Autodesk Inventor part; units mm, degrees
(part 2 of 2)
sketch "Sketch39" plane through (0, 15, 0) normal (0, 1, 0) x (1, 0, 0)
  circle A0 centre (1.2218, -51.2393) radius 1.65 projected
  circle A1 centre (75, -20) radius 1.65 projected
  circle A2 centre (75, 20) radius 1.65 projected
  circle A3 centre (1.2218, 51.2393) radius 1.65 projected
  circle A4 centre (50, -41.2393) radius 1.65 projected
  circle A5 centre (50, 41.4252) radius 1.65 projected
  arc A6 (-52, -67.2384) -> (-18.7782, -82.8998) centre (0, 0) ccw projected
  line L0 (-52, -67.2384) -> (-52, 67.2384) projected
  arc A7 (-18.7782, 82.8998) -> (-52, 67.2384) centre (0, 0) ccw projected
  line L1 (-18.7782, 82.8998) -> (-18.7782, -82.8998) projected
  circle A8 centre (-8.7782, 43.7683) radius 1.6079 projected
  circle A9 centre (-8.778, -38.7103) radius 1.6079 projected
  circle A10 centre (1.2218, -41.2393) radius 1.65 projected
  circle A11 centre (1.2218, 41.2393) radius 1.65 projected
  line L2 (-28.2493, 88.8562) -> (-25.8738, 89.6874) projected
  line L3 (-25.8738, 89.6874) -> (-24.5197, 85.8175) projected
  line L4 (-24.5197, 85.8175) -> (-34.3361, 82.3826) projected
  line L5 (-34.3361, 82.3826) -> (-35.6902, 86.2525) projected
  line L6 (-35.6902, 86.2525) -> (-33.3147, 87.0837) projected
  arc A12 (-28.2493, 88.8562) -> (-33.3147, 87.0837) centre (-30.4187, 86.9317) ccw projected
  line L7 (30.0353, 88.2685) -> (32.4402, 87.5267) projected
  line L8 (32.4402, 87.5267) -> (31.2317, 83.6088) projected
  line L9 (31.2317, 83.6088) -> (21.2937, 86.6743) projected
  line L10 (21.2937, 86.6743) -> (22.5022, 90.5921) projected
  line L11 (22.5022, 90.5921) -> (24.9071, 89.8503) projected
  arc A13 (30.0353, 88.2685) -> (24.9071, 89.8503) centre (27.147, 88.0083) ccw projected
  line L12 (79.29, 49.114) -> (80.6765, 47.0136) projected
  line L13 (80.6765, 47.0136) -> (77.2547, 44.7549) projected
  line L14 (77.2547, 44.7549) -> (71.5254, 53.4345) projected
  line L15 (71.5254, 53.4345) -> (74.9472, 55.6931) projected
  line L16 (74.9472, 55.6931) -> (76.3336, 53.5927) projected
  arc A14 (79.29, 49.114) -> (76.3336, 53.5927) centre (76.8938, 50.7474) ccw projected
  line L17 (93.2, -2.6833) -> (93.2, -5.2) projected
  line L18 (93.2, -5.2) -> (89.1, -5.2) projected
  line L19 (89.1, -5.2) -> (89.1, 5.2) projected
  line L20 (89.1, 5.2) -> (93.2, 5.2) projected
  line L21 (93.2, 5.2) -> (93.2, 2.6833) projected
  arc A15 (93.2, -2.6833) -> (93.2, 2.6833) centre (92.1, 0) ccw projected
  line L22 (76.6444, -54.0482) -> (75.2579, -56.1486) projected
  line L23 (75.2579, -56.1486) -> (71.8362, -53.8899) projected
  line L24 (71.8362, -53.8899) -> (77.5655, -45.2103) projected
  line L25 (77.5655, -45.2103) -> (80.9873, -47.469) projected
  line L26 (80.9873, -47.469) -> (79.6008, -49.5694) projected
  arc A16 (76.6444, -54.0482) -> (79.6008, -49.5694) centre (77.2046, -51.2028) ccw projected
  line L27 (24.9071, -89.8503) -> (22.5022, -90.5921) projected
  line L28 (22.5022, -90.5921) -> (21.2937, -86.6743) projected
  line L29 (21.2937, -86.6743) -> (31.2317, -83.6088) projected
  line L30 (31.2317, -83.6088) -> (32.4402, -87.5267) projected
  line L31 (32.4402, -87.5267) -> (30.0353, -88.2685) projected
  arc A17 (24.9071, -89.8503) -> (30.0353, -88.2685) centre (27.147, -88.0083) ccw projected
  line L32 (-33.3147, -87.0837) -> (-35.6902, -86.2525) projected
  line L33 (-35.6902, -86.2525) -> (-34.3361, -82.3826) projected
  line L34 (-34.3361, -82.3826) -> (-24.5197, -85.8175) projected
  line L35 (-24.5197, -85.8175) -> (-25.8738, -89.6874) projected
  line L36 (-25.8738, -89.6874) -> (-28.2493, -88.8562) projected
  arc A18 (-33.3147, -87.0837) -> (-28.2493, -88.8562) centre (-30.4187, -86.9317) ccw projected
  line L37 (-68.5526, -41.4252) -> (-65.0019, -39.3752) projected
  line L38 (-65.0019, -39.3752) -> (-59.8019, -48.3819) projected
  line L39 (-59.8019, -48.3819) -> (-63.3526, -50.4319) projected
  line L40 (-63.3526, -50.4319) -> (-64.611, -48.2524) projected
  arc A19 (-67.2943, -43.6048) -> (-64.611, -48.2524) centre (-65, -45.3786) ccw projected
  line L41 (-67.2943, -43.6048) -> (-68.5526, -41.4252) projected
  line L42 (-64.7167, 27.997) -> (-60.7564, 26.9359) projected
  line L43 (-60.7564, 26.9359) -> (-63.4481, 16.8902) projected
  line L44 (-63.4481, 16.8902) -> (-67.4084, 17.9514) projected
  line L45 (-67.4084, 17.9514) -> (-66.757, 20.3823) projected
  arc A20 (-65.368, 25.5661) -> (-66.757, 20.3823) centre (-65, 22.6895) ccw projected
  line L46 (-65.368, 25.5661) -> (-64.7167, 27.997) projected
  line L47 (-66.1, 5.2) -> (-62, 5.2) projected
  line L48 (-62, 5.2) -> (-62, -5.2) projected
  line L49 (-62, -5.2) -> (-66.1, -5.2) projected
  line L50 (-66.1, -5.2) -> (-66.1, -2.6833) projected
  arc A21 (-66.1, 2.6833) -> (-66.1, -2.6833) centre (-65, 0) ccw projected
  line L51 (-66.1, 2.6833) -> (-66.1, 5.2) projected
  line L52 (-67.4084, -17.9514) -> (-63.4481, -16.8902) projected
  line L53 (-63.4481, -16.8902) -> (-60.7564, -26.9359) projected
  line L54 (-60.7564, -26.9359) -> (-64.7167, -27.997) projected
  line L55 (-64.7167, -27.997) -> (-65.368, -25.5661) projected
  arc A22 (-66.757, -20.3823) -> (-65.368, -25.5661) centre (-65, -22.6895) ccw projected
  line L56 (-66.757, -20.3823) -> (-67.4084, -17.9514) projected
  line L57 (-63.3526, 50.4319) -> (-59.8019, 48.3819) projected
  line L58 (-59.8019, 48.3819) -> (-65.0019, 39.3752) projected
  line L59 (-65.0019, 39.3752) -> (-68.5526, 41.4252) projected
  line L60 (-68.5526, 41.4252) -> (-67.2943, 43.6048) projected
  arc A23 (-64.611, 48.2524) -> (-67.2943, 43.6048) centre (-65, 45.3786) ccw projected
  line L61 (-64.611, 48.2524) -> (-63.3526, 50.4319) projected
  line L62 (-60.862, -70.775) -> (-58.3661, -67.5222) projected
  line L63 (-58.3661, -67.5222) -> (-50.1152, -73.8533) projected
  line L64 (-50.1152, -73.8533) -> (-52.6111, -77.1061) projected
  line L65 (-52.6111, -77.1061) -> (-54.6078, -75.574) projected
  arc A24 (-58.8654, -72.3071) -> (-54.6078, -75.574) centre (-56.0669, -73.0678) ccw projected
  line L66 (-58.8654, -72.3071) -> (-60.862, -70.775) projected
  line L67 (-4.4255, -93.1335) -> (-6.9418, -93.0865) projected
  line L68 (-6.9418, -93.0865) -> (-6.8652, -88.9872) projected
  line L69 (-6.8652, -88.9872) -> (3.533, -89.1817) projected
  line L70 (3.533, -89.1817) -> (3.4564, -93.2809) projected
  line L71 (3.4564, -93.2809) -> (0.9401, -93.2339) projected
  arc A25 (-4.4255, -93.1335) -> (0.9401, -93.2339) centre (-1.7222, -92.0839) ccw projected
  line L72 (51.7438, -77.563) -> (49.6912, -79.0194) projected
  line L73 (49.6912, -79.0194) -> (47.3187, -75.6756) projected
  line L74 (47.3187, -75.6756) -> (55.8005, -69.6574) projected
  line L75 (55.8005, -69.6574) -> (58.1731, -73.0012) projected
  line L76 (58.1731, -73.0012) -> (56.1205, -74.4575) projected
  arc A26 (51.7438, -77.563) -> (56.1205, -74.4575) centre (53.2956, -75.1132) ccw projected
  line L77 (87.6914, -31.6805) -> (86.9048, -34.0711) projected
  line L78 (86.9048, -34.0711) -> (83.0102, -32.7896) projected
  line L79 (83.0102, -32.7896) -> (86.2609, -22.9107) projected
  line L80 (86.2609, -22.9107) -> (90.1555, -24.1922) projected
  line L81 (90.1555, -24.1922) -> (89.3689, -26.5829) projected
  arc A27 (87.6914, -31.6805) -> (89.3689, -26.5829) centre (87.4853, -28.7879) ccw projected
  line L82 (89.3689, 26.5829) -> (90.1555, 24.1922) projected
  line L83 (90.1555, 24.1922) -> (86.2609, 22.9107) projected
  line L84 (86.2609, 22.9107) -> (83.0102, 32.7896) projected
  line L85 (83.0102, 32.7896) -> (86.9048, 34.0711) projected
  line L86 (86.9048, 34.0711) -> (87.6914, 31.6805) projected
  arc A28 (89.3689, 26.5829) -> (87.6914, 31.6805) centre (87.4853, 28.7879) ccw projected
  line L87 (56.1205, 74.4575) -> (58.1731, 73.0012) projected
  line L88 (58.1731, 73.0012) -> (55.8005, 69.6574) projected
  line L89 (55.8005, 69.6574) -> (47.3187, 75.6756) projected
  line L90 (47.3187, 75.6756) -> (49.6912, 79.0194) projected
  line L91 (49.6912, 79.0194) -> (51.7438, 77.563) projected
  arc A29 (56.1205, 74.4575) -> (51.7438, 77.563) centre (53.2956, 75.1132) ccw projected
  line L92 (0.9401, 93.2339) -> (3.4564, 93.2809) projected
  line L93 (3.4564, 93.2809) -> (3.533, 89.1817) projected
  line L94 (3.533, 89.1817) -> (-6.8652, 88.9872) projected
  line L95 (-6.8652, 88.9872) -> (-6.9418, 93.0865) projected
  line L96 (-6.9418, 93.0865) -> (-4.4255, 93.1335) projected
  arc A30 (0.9401, 93.2339) -> (-4.4255, 93.1335) centre (-1.7222, 92.0839) ccw projected
  line L97 (-54.6078, 75.574) -> (-52.6111, 77.1061) projected
  line L98 (-52.6111, 77.1061) -> (-50.1152, 73.8533) projected
  line L99 (-50.1152, 73.8533) -> (-58.3661, 67.5222) projected
  line L100 (-58.3661, 67.5222) -> (-60.862, 70.775) projected
  line L101 (-60.862, 70.775) -> (-58.8654, 72.3071) projected
  arc A31 (-54.6078, 75.574) -> (-58.8654, 72.3071) centre (-56.0669, 73.0678) ccw projected
  circle A32 centre (-57, -37.4412) radius 1.25 projected
  circle A33 centre (-57, 37.4412) radius 1.25 projected
  circle A34 centre (-69.5802, -56.8899) radius 3 projected
  circle A35 centre (-69.5802, 56.8899) radius 3 projected
  circle A36 centre (71.6532, 61.1111) radius 3 projected
  circle A37 centre (71.6532, -61.1111) radius 3 projected
  line L102 (6.2218, -84.772) -> (6.2218, 84.772) projected
  arc A38 (45, 72.111) -> (6.2218, 84.772) centre (0, 0) ccw projected
  line L103 (45, 72.111) -> (45, -72.111) projected
  arc A39 (6.2218, -84.772) -> (45, -72.111) centre (0, 0) ccw projected
  arc A40 (-85, -52.6783) -> (-85, 52.6783) centre (0, 0) ccw projected
  line L104 (-18.7782, 82.8998) -> (6.2218, 82.8998)
  line L105 (6.2218, -84.772) -> (6.2218, 84.772) projected
  line L106 (-18.7782, 83.6088) -> (-18.7782, 63.6088)
  line L107 (-18.7782, 82.8998) -> (-18.7782, -82.8998) projected
  line L108 (-18.7782, 63.6088) -> (6.2218, 63.6088)
  line L109 (6.2218, 63.6088) -> (6.2218, 82.8998)
  line L110 (-85, 52.6783) -> (-85, 47.6783) projected
  line L111 (-85, -47.6783) -> (-85, -52.6783) projected
  line L112 (-70, 0) -> (-85, -47.6783) projected
  line L113 (-85, 47.6783) -> (-70, 0) projected
  dimension "d78" = 10.4
  dimension "d79" = 4.1
  dimension "d243" = 20
  constraints: 8 end point, 3 point on line, 1 collinear, 1 horizontal, 1 perpendicular
  measures "d243" distance of L106.start L106.end
extrude "Extrusion37" add sketch "Sketch39" along normal blind 25 contours L1 L104 L102 L108
sketch "Sketch40" plane through (-18.7782, 15, -63.6088) normal (0, 0, 1) x (1, 0, 0)
  line L0 (0, -5) -> (0, 0) projected
  line L1 (2.25, 1) -> (22.75, 1)
  line L2 (22.75, 1) -> (22.75, 24)
  line L3 (22.75, 24) -> (2.25, 24)
  line L4 (2.25, 24) -> (2.25, 1)
  line L5 (2.25, 1) -> (22.75, 24) construction
  line L6 (22.75, 1) -> (2.25, 24) construction
  line L7 (25, 0) -> (25, 25) projected
  point P0 (18.7782, -15)
  point P1 (0, 25)
  point P2 (12.5, 12.5)
  dimension "d246" = 20.5
  dimension "d247" = 23
  constraints: 12 end point, 2 midpoint, 2 parallel, 2 perpendicular
  measures "d246" distance of L1.start L1.end
  measures "d247" distance of L2.end L1.end
extrude "Extrusion38" cut sketch "Sketch40" against normal blind 5
sketch "Sketch41" plane through (-18.7782, 15, -68.6088) normal (0, 0, 1) x (1, 0, 0)
  line L0 (22.75, 1) -> (2.25, 1) projected
  line L1 (22.75, 24) -> (22.75, 1) projected
  line L2 (2.25, 24) -> (22.75, 24) projected
  line L3 (2.25, 1) -> (2.25, 24) projected
  line L4 (22.75, 1) -> (2.25, 1)
  circle A0 centre (13.7, 12.5) radius 8.5
  line L5 (22.75, 1) -> (22.45, 1)
  line L6 (22.75, 1) -> (2.25, 1) projected
  line L7 (22.45, 1) -> (22.45, 1.45)
  line L8 (22.45, 1.45) -> (20, 1.45)
  line L9 (20, 1.45) -> (20, 3.9)
  line L10 (20, 3.9) -> (7.4, 3.9)
  line L11 (13.7, 3.9) -> (13.7, 12.5)
  line L12 (13.7, 3.9) -> (22.3, 3.9) construction
  point P0 (18.7782, -15)
  dimension "d250" = 17
  dimension "d272" = 0.3
  dimension "d273" = 0.45
  dimension "d274" = 2.45
  dimension "d275" = 2.45
  dimension "d276" = 12.6
  dimension "d277" = 90
  constraints: 16 end point, 5 perpendicular, 1 centre point, 1 collinear, 1 horizontal, 1 midpoint, 1 point on line
  measures "d250" diameter of A0
  measures "d272" distance of L0.start L5.end
  measures "d273" distance of L5.end L7.end
  measures "d274" distance of L7.end L8.end
  measures "d275" distance of L8.end L9.end
  measures "d276" distance of L9.end L10.end
  measures "d277" angle of L12 L11
extrude "Extrusion39" cut sketch "Sketch41" against normal blind 48.5 contours A0
sketch "Sketch42" plane through (-18.7782, 15, -68.6088) normal (0, 0, 1) x (1, 0, 0)
  circle A0 centre (13.7, 12.5) radius 8.5 projected
  line L0 (22.75, 1) -> (2.25, 1) projected
  line L1 (22.75, 24) -> (22.75, 1) projected
  line L2 (2.25, 24) -> (22.75, 24) projected
  line L3 (2.25, 1) -> (2.25, 24) projected
  line L4 (22.75, 1) -> (22.75, 1.45)
  line L5 (22.75, 24) -> (22.75, 1) projected
  line L6 (22.75, 1.45) -> (22.75, 3.99)
  line L7 (2.25, 1) -> (2.25, 24) projected
  line L8 (2.25, 4) -> (2.55, 4)
  line L9 (22.75, 24) -> (22.75, 23.55)
  line L10 (22.45, 1.45) -> (2.55, 1.45)
  line L11 (2.55, 1.45) -> (2.55, 23.55)
  line L12 (2.55, 23.55) -> (22.45, 23.55)
  line L13 (22.45, 23.55) -> (22.45, 1.45)
  line L14 (22.45, 1.45) -> (22.45, 3.99)
  line L15 (22.45, 3.99) -> (19.91, 3.99)
  line L16 (19.91, 3.99) -> (7.31, 3.99)
  line L17 (7.31, 3.99) -> (7.31, 20.99)
  line L18 (7.31, 20.99) -> (19.91, 20.99)
  circle A1 centre (7.31, 20.99) radius 1.25
  circle A2 centre (19.91, 3.99) radius 1.25
  point P0 (18.7782, -15)
  dimension "d253" = 0.45
  dimension "d254" = 2.54
  dimension "d261" = 0.3
  dimension "d262" = 0.45
  dimension "d263" = 0.3
  dimension "d264" = 2.54
  dimension "d265" = 2.54
  dimension "d266" = 12.6
  dimension "d267" = 17
  dimension "d268" = 2.5
  dimension "d269" = 2.5
  constraints: 26 end point, 6 perpendicular, 6 point on line, 2 centre point, 2 coincident, 1 parallel
  measures "d253" distance of L0.start L4.end
  measures "d254" distance of L4.end L6.end
  measures "d261" distance of L8.start L8.end
  measures "d262" distance of L1.start L9.end
  measures "d263" distance of L4.end L10.start
  measures "d264" distance of L10.start L14.end
  measures "d265" distance of L14.end L15.end
  measures "d266" distance of L15.end L16.end
  measures "d267" distance of L16.end L17.end
  measures "d268" diameter of A1
  measures "d269" diameter of A2
extrude "Extrusion40" cut sketch "Sketch42" against normal blind 10 contours A1 L17 L18 | L18 L17 A1 | A2 L16 L15 | L15 L16 A2
sketch "Sketch43" plane through (0, 15, 0) normal (0, 1, 0) x (1, 0, 0)
  line L0 (-18.7782, -82.8998) -> (6.2218, -82.8998)
  line L1 (6.2218, -84.772) -> (6.2218, 63.6088) projected
  line L2 (-18.7782, -82.8998) -> (-18.7782, -62.8998)
  line L3 (-18.7782, -82.8998) -> (-18.7782, 82.8998) projected
  line L4 (6.2218, -82.8998) -> (6.2218, -62.8998)
  line L5 (6.2218, -62.8998) -> (-18.7782, -62.8998)
  line L6 (-18.7782, 63.6088) -> (-18.7782, -82.8998) projected
  point P0 (0, 0)
  dimension "d278" = 20
  constraints: 8 end point, 3 point on line, 1 horizontal, 1 perpendicular
  measures "d278" distance of L0.start L2.end
extrude "Extrusion41" add sketch "Sketch43" along normal blind 25
sketch "Sketch44" plane through (6.2218, 15, 62.8998) normal (0, 0, -1) x (-1, 0, 0)
  line L0 (2.25, 1) -> (22.75, 1) projected
  line L1 (2.25, 24) -> (2.25, 1) projected
  line L2 (22.75, 24) -> (2.25, 24) projected
  line L3 (22.75, 1) -> (22.75, 24) projected
  point P0 (6.2218, -15)
extrude "Extrusion42" cut sketch "Sketch44" against normal blind 5
sketch "Sketch45" plane through (6.2218, 15, 67.8998) normal (0, 0, -1) x (-1, 0, 0)
  line L0 (22.75, 1) -> (2.25, 1) projected
  line L1 (22.75, 24) -> (22.75, 1) projected
  line L2 (2.25, 24) -> (22.75, 24) projected
  line L3 (2.25, 1) -> (2.25, 24) projected
  line L4 (22.75, 1) -> (22.75, 1.45)
  line L5 (22.75, 24) -> (22.75, 1) projected
  line L6 (22.45, 1.45) -> (24.9, 1.45) construction
  circle A0 centre (13.7, 12.5) radius 8.5
  circle A1 centre (20, 3.9) radius 1.25
  circle A2 centre (7.4, 20.9) radius 1.25
  point P0 (6.2218, -15)
  dimension "d283" = 0.45
  dimension "d284" = 0.3
  dimension "d292" = 2.5
  dimension "d295" = 2.5
  constraints: 4 end point, 3 centre point, 1 horizontal, 1 point on line
  measures "d283" distance of L0.start L4.end
  measures "d284" distance of L4.end L6.start
  measures "d292" diameter of A1
  measures "d295" diameter of A2
extrude "Extrusion43" cut sketch "Sketch45" against normal through all contours A0
sketch "Sketch46" plane through (6.2218, 15, 67.8998) normal (0, 0, -1) x (-1, 0, 0)
  line L0 (22.75, 1) -> (2.25, 1)
  line L1 (22.75, 24) -> (22.75, 1)
  line L2 (2.25, 24) -> (22.75, 24)
  line L3 (2.25, 1) -> (2.25, 24)
  line L4 (22.75, 1) -> (22.75, 1.45)
  line L5 (22.75, 24) -> (22.75, 1)
  line L6 (22.45, 1.45) -> (24.9, 1.45) construction
  circle A0 centre (13.7, 12.5) radius 8.5
  circle A1 centre (20, 3.9) radius 1.25
  circle A2 centre (7.4, 20.9) radius 1.25
  point P0 (6.2218, -15)
  dimension "d298" = 0.45
  dimension "d299" = 0.3
  dimension "d300" = 2.5
  dimension "d301" = 2.5
  constraints: 14 end point, 3 centre point, 1 horizontal, 1 point on line
  measures "d298" distance of L0.start L4.end
  measures "d299" distance of L4.end L6.start
  measures "d300" diameter of A1
  measures "d301" diameter of A2
extrude "Extrusion44" cut sketch "Sketch46" against normal blind 10 contours A1 | A2
sketch "Sketch47" plane through (0, 15, 0) normal (0, 1, 0) x (1, 0, 0)
  circle A0 centre (75, -20) radius 1.65 projected
  circle A1 centre (75, 20) radius 1.65 projected
  circle A2 centre (50, -41.2393) radius 1.65 projected
  circle A3 centre (50, 41.4252) radius 1.65 projected
  line L0 (-28.2493, 88.8562) -> (-25.8738, 89.6874) projected
  line L1 (-25.8738, 89.6874) -> (-24.5197, 85.8175) projected
  line L2 (-24.5197, 85.8175) -> (-34.3361, 82.3826) projected
  line L3 (-34.3361, 82.3826) -> (-35.6902, 86.2525) projected
  line L4 (-35.6902, 86.2525) -> (-33.3147, 87.0837) projected
  arc A4 (-28.2493, 88.8562) -> (-33.3147, 87.0837) centre (-30.4187, 86.9317) ccw projected
  line L5 (30.0353, 88.2685) -> (32.4402, 87.5267) projected
  line L6 (32.4402, 87.5267) -> (31.2317, 83.6088) projected
  line L7 (31.2317, 83.6088) -> (21.2937, 86.6743) projected
  line L8 (21.2937, 86.6743) -> (22.5022, 90.5921) projected
  line L9 (22.5022, 90.5921) -> (24.9071, 89.8503) projected
  arc A5 (30.0353, 88.2685) -> (24.9071, 89.8503) centre (27.147, 88.0083) ccw projected
  line L10 (79.29, 49.114) -> (80.6765, 47.0136) projected
  line L11 (80.6765, 47.0136) -> (77.2547, 44.7549) projected
  line L12 (77.2547, 44.7549) -> (71.5254, 53.4345) projected
  line L13 (71.5254, 53.4345) -> (74.9472, 55.6931) projected
  line L14 (74.9472, 55.6931) -> (76.3336, 53.5927) projected
  arc A6 (79.29, 49.114) -> (76.3336, 53.5927) centre (76.8938, 50.7474) ccw projected
  line L15 (93.2, -2.6833) -> (93.2, -5.2) projected
  line L16 (93.2, -5.2) -> (89.1, -5.2) projected
  line L17 (89.1, -5.2) -> (89.1, 5.2) projected
  line L18 (89.1, 5.2) -> (93.2, 5.2) projected
  line L19 (93.2, 5.2) -> (93.2, 2.6833) projected
  arc A7 (93.2, -2.6833) -> (93.2, 2.6833) centre (92.1, 0) ccw projected
  line L20 (76.6444, -54.0482) -> (75.2579, -56.1486) projected
  line L21 (75.2579, -56.1486) -> (71.8362, -53.8899) projected
  line L22 (71.8362, -53.8899) -> (77.5655, -45.2103) projected
  line L23 (77.5655, -45.2103) -> (80.9873, -47.469) projected
  line L24 (80.9873, -47.469) -> (79.6008, -49.5694) projected
  arc A8 (76.6444, -54.0482) -> (79.6008, -49.5694) centre (77.2046, -51.2028) ccw projected
  line L25 (24.9071, -89.8503) -> (22.5022, -90.5921) projected
  line L26 (22.5022, -90.5921) -> (21.2937, -86.6743) projected
  line L27 (21.2937, -86.6743) -> (31.2317, -83.6088) projected
  line L28 (31.2317, -83.6088) -> (32.4402, -87.5267) projected
  line L29 (32.4402, -87.5267) -> (30.0353, -88.2685) projected
  arc A9 (24.9071, -89.8503) -> (30.0353, -88.2685) centre (27.147, -88.0083) ccw projected
  line L30 (-33.3147, -87.0837) -> (-35.6902, -86.2525) projected
  line L31 (-35.6902, -86.2525) -> (-34.3361, -82.3826) projected
  line L32 (-34.3361, -82.3826) -> (-24.5197, -85.8175) projected
  line L33 (-24.5197, -85.8175) -> (-25.8738, -89.6874) projected
  line L34 (-25.8738, -89.6874) -> (-28.2493, -88.8562) projected
  arc A10 (-33.3147, -87.0837) -> (-28.2493, -88.8562) centre (-30.4187, -86.9317) ccw projected
  line L35 (-68.5526, -41.4252) -> (-65.0019, -39.3752) projected
  line L36 (-65.0019, -39.3752) -> (-59.8019, -48.3819) projected
  line L37 (-59.8019, -48.3819) -> (-63.3526, -50.4319) projected
  line L38 (-63.3526, -50.4319) -> (-64.611, -48.2524) projected
  arc A11 (-67.2943, -43.6048) -> (-64.611, -48.2524) centre (-65, -45.3786) ccw projected
  line L39 (-67.2943, -43.6048) -> (-68.5526, -41.4252) projected
  line L40 (-64.7167, 27.997) -> (-60.7564, 26.9359) projected
  line L41 (-60.7564, 26.9359) -> (-63.4481, 16.8902) projected
  line L42 (-63.4481, 16.8902) -> (-67.4084, 17.9514) projected
  line L43 (-67.4084, 17.9514) -> (-66.757, 20.3823) projected
  arc A12 (-65.368, 25.5661) -> (-66.757, 20.3823) centre (-65, 22.6895) ccw projected
  line L44 (-65.368, 25.5661) -> (-64.7167, 27.997) projected
  line L45 (-66.1, 5.2) -> (-62, 5.2) projected
  line L46 (-62, 5.2) -> (-62, -5.2) projected
  line L47 (-62, -5.2) -> (-66.1, -5.2) projected
  line L48 (-66.1, -5.2) -> (-66.1, -2.6833) projected
  arc A13 (-66.1, 2.6833) -> (-66.1, -2.6833) centre (-65, 0) ccw projected
  line L49 (-66.1, 2.6833) -> (-66.1, 5.2) projected
  line L50 (-67.4084, -17.9514) -> (-63.4481, -16.8902) projected
  line L51 (-63.4481, -16.8902) -> (-60.7564, -26.9359) projected
  line L52 (-60.7564, -26.9359) -> (-64.7167, -27.997) projected
  line L53 (-64.7167, -27.997) -> (-65.368, -25.5661) projected
  arc A14 (-66.757, -20.3823) -> (-65.368, -25.5661) centre (-65, -22.6895) ccw projected
  line L54 (-66.757, -20.3823) -> (-67.4084, -17.9514) projected
  line L55 (-63.3526, 50.4319) -> (-59.8019, 48.3819) projected
  line L56 (-59.8019, 48.3819) -> (-65.0019, 39.3752) projected
  line L57 (-65.0019, 39.3752) -> (-68.5526, 41.4252) projected
  line L58 (-68.5526, 41.4252) -> (-67.2943, 43.6048) projected
  arc A15 (-64.611, 48.2524) -> (-67.2943, 43.6048) centre (-65, 45.3786) ccw projected
  line L59 (-64.611, 48.2524) -> (-63.3526, 50.4319) projected
  line L60 (-60.862, -70.775) -> (-58.3661, -67.5222) projected
  line L61 (-58.3661, -67.5222) -> (-50.1152, -73.8533) projected
  line L62 (-50.1152, -73.8533) -> (-52.6111, -77.1061) projected
  line L63 (-52.6111, -77.1061) -> (-54.6078, -75.574) projected
  arc A16 (-58.8654, -72.3071) -> (-54.6078, -75.574) centre (-56.0669, -73.0678) ccw projected
  line L64 (-58.8654, -72.3071) -> (-60.862, -70.775) projected
  line L65 (-4.4255, -93.1335) -> (-6.9418, -93.0865) projected
  line L66 (-6.9418, -93.0865) -> (-6.8652, -88.9872) projected
  line L67 (-6.8652, -88.9872) -> (3.533, -89.1817) projected
  line L68 (3.533, -89.1817) -> (3.4564, -93.2809) projected
  line L69 (3.4564, -93.2809) -> (0.9401, -93.2339) projected
  arc A17 (-4.4255, -93.1335) -> (0.9401, -93.2339) centre (-1.7222, -92.0839) ccw projected
  line L70 (51.7438, -77.563) -> (49.6912, -79.0194) projected
  line L71 (49.6912, -79.0194) -> (47.3187, -75.6756) projected
  line L72 (47.3187, -75.6756) -> (55.8005, -69.6574) projected
  line L73 (55.8005, -69.6574) -> (58.1731, -73.0012) projected
  line L74 (58.1731, -73.0012) -> (56.1205, -74.4575) projected
  arc A18 (51.7438, -77.563) -> (56.1205, -74.4575) centre (53.2956, -75.1132) ccw projected
  line L75 (87.6914, -31.6805) -> (86.9048, -34.0711) projected
  line L76 (86.9048, -34.0711) -> (83.0102, -32.7896) projected
  line L77 (83.0102, -32.7896) -> (86.2609, -22.9107) projected
  line L78 (86.2609, -22.9107) -> (90.1555, -24.1922) projected
  line L79 (90.1555, -24.1922) -> (89.3689, -26.5829) projected
  arc A19 (87.6914, -31.6805) -> (89.3689, -26.5829) centre (87.4853, -28.7879) ccw projected
  line L80 (89.3689, 26.5829) -> (90.1555, 24.1922) projected
  line L81 (90.1555, 24.1922) -> (86.2609, 22.9107) projected
  line L82 (86.2609, 22.9107) -> (83.0102, 32.7896) projected
  line L83 (83.0102, 32.7896) -> (86.9048, 34.0711) projected
  line L84 (86.9048, 34.0711) -> (87.6914, 31.6805) projected
  arc A20 (89.3689, 26.5829) -> (87.6914, 31.6805) centre (87.4853, 28.7879) ccw projected
  line L85 (56.1205, 74.4575) -> (58.1731, 73.0012) projected
  line L86 (58.1731, 73.0012) -> (55.8005, 69.6574) projected
  line L87 (55.8005, 69.6574) -> (47.3187, 75.6756) projected
  line L88 (47.3187, 75.6756) -> (49.6912, 79.0194) projected
  line L89 (49.6912, 79.0194) -> (51.7438, 77.563) projected
  arc A21 (56.1205, 74.4575) -> (51.7438, 77.563) centre (53.2956, 75.1132) ccw projected
  line L90 (0.9401, 93.2339) -> (3.4564, 93.2809) projected
  line L91 (3.4564, 93.2809) -> (3.533, 89.1817) projected
  line L92 (3.533, 89.1817) -> (-6.8652, 88.9872) projected
  line L93 (-6.8652, 88.9872) -> (-6.9418, 93.0865) projected
  line L94 (-6.9418, 93.0865) -> (-4.4255, 93.1335) projected
  arc A22 (0.9401, 93.2339) -> (-4.4255, 93.1335) centre (-1.7222, 92.0839) ccw projected
  line L95 (-54.6078, 75.574) -> (-52.6111, 77.1061) projected
  line L96 (-52.6111, 77.1061) -> (-50.1152, 73.8533) projected
  line L97 (-50.1152, 73.8533) -> (-58.3661, 67.5222) projected
  line L98 (-58.3661, 67.5222) -> (-60.862, 70.775) projected
  line L99 (-60.862, 70.775) -> (-58.8654, 72.3071) projected
  arc A23 (-54.6078, 75.574) -> (-58.8654, 72.3071) centre (-56.0669, 73.0678) ccw projected
  circle A24 centre (-57, -37.4412) radius 1.25 projected
  circle A25 centre (-57, 37.4412) radius 1.25 projected
  circle A26 centre (-69.5802, -56.8899) radius 3 projected
  circle A27 centre (-69.5802, 56.8899) radius 3 projected
  circle A28 centre (71.6532, 61.1111) radius 3 projected
  circle A29 centre (71.6532, -61.1111) radius 3 projected
  arc A30 (-85, -52.6783) -> (-85, 52.6783) centre (0, 0) ccw projected
  line L100 (6.2218, -82.8998) -> (-18.7782, -82.8998) projected
  arc A31 (-52, -67.2384) -> (-18.7782, -82.8998) centre (0, 0) ccw projected
  line L101 (-52, -67.2384) -> (-52, 67.2384) projected
  arc A32 (-18.7782, 82.8998) -> (-52, 67.2384) centre (0, 0) ccw projected
  line L102 (-18.7782, 82.8998) -> (6.2218, 82.8998) projected
  line L103 (6.2218, 82.8998) -> (6.2218, 84.772) projected
  arc A33 (45, 72.111) -> (6.2218, 84.772) centre (0, 0) ccw projected
  line L104 (45, 72.111) -> (45, -72.111) projected
  arc A34 (6.2218, -84.772) -> (45, -72.111) centre (0, 0) ccw projected
  line L105 (6.2218, -84.772) -> (6.2218, -82.8998) projected
  line L106 (82, 0) -> (82, -12.5)
  line L107 (82, -12.5) -> (62, -12.5)
  line L108 (62, -12.5) -> (62, 12.5)
  line L109 (62, 12.5) -> (82, 12.5)
  line L110 (82, 12.5) -> (82, 0)
  line L111 (-85, 52.6783) -> (-85, 47.6783) projected
  line L112 (-85, -47.6783) -> (-85, -52.6783) projected
  line L113 (-70, 0) -> (-85, -47.6783) projected
  line L114 (-85, 47.6783) -> (-70, 0) projected
  dimension "d306" = 20
  dimension "d307" = 25
  constraints: 10 end point, 4 perpendicular, 1 point on line, 1 vertical
  measures "d306" distance of L106.end L107.end
  measures "d307" distance of L107.end L108.end
extrude "Extrusion45" add sketch "Sketch47" along normal blind 25 contours L106 L107 L108 L109 L110
sketch "Sketch48" plane through (62, 15, -12.5) normal (-1, 0, 0) x (0, 0, 1)
  line L0 (25, 0) -> (0, 0) projected
  line L1 (25, 0) -> (25, 25) projected
  line L2 (0, 25) -> (25, 25) projected
  line L3 (0, 0) -> (0, 25) projected
  line L4 (2.25, 24) -> (2.25, 1)
  line L5 (2.25, 1) -> (22.75, 1)
  line L6 (22.75, 1) -> (22.75, 24)
  line L7 (22.75, 24) -> (2.25, 24)
  line L8 (2.25, 24) -> (22.75, 1) construction
  line L9 (2.25, 1) -> (22.75, 24) construction
  point P0 (12.5, -15)
  point P1 (12.5, 12.5)
  dimension "d310" = 23
  dimension "d311" = 20.5
  constraints: 12 end point, 2 midpoint, 2 parallel, 1 perpendicular, 1 vertical
  measures "d310" distance of L4.start L4.end
  measures "d311" distance of L5.end L4.end
extrude "Extrusion46" cut sketch "Sketch48" against normal blind 5 contours L7 L6 L5 L4
sketch "Sketch49" plane through (67, 15, -12.5) normal (-1, 0, 0) x (0, 0, 1)
  line L0 (2.25, 1) -> (2.25, 24) projected
  line L1 (22.75, 1) -> (2.25, 1) projected
  line L2 (22.75, 24) -> (22.75, 1) projected
  line L3 (2.25, 24) -> (22.75, 24) projected
  line L4 (22.75, 1) -> (22.45, 1)
  circle A0 centre (13.7, 12.5) radius 8.5
  circle A1 centre (7.4, 20.9) radius 1.25
  circle A2 centre (20, 3.9) radius 1.25
  point P0 (12.5, -15)
  dimension "d314" = 0.3
  dimension "d320" = 17
  dimension "d321" = 2.5
  dimension "d322" = 2.5
  constraints: 3 centre point, 2 end point, 1 point on line
  measures "d314" distance of L1.start L4.end
  measures "d320" diameter of A0
  measures "d321" diameter of A1
  measures "d322" diameter of A2
extrude "Extrusion47" cut sketch "Sketch49" against normal through all contours A0
sketch "Sketch50" plane through (67, 15, -12.5) normal (-1, 0, 0) x (0, 0, 1)
  line L0 (2.25, 1) -> (2.25, 24)
  line L1 (22.75, 1) -> (2.25, 1)
  line L2 (22.75, 24) -> (22.75, 1)
  line L3 (2.25, 24) -> (22.75, 24)
  line L4 (22.75, 1) -> (22.45, 1)
  circle A0 centre (13.7, 12.5) radius 8.5
  circle A1 centre (7.4, 20.9) radius 1.25
  circle A2 centre (20, 3.9) radius 1.25
  point P0 (12.5, -15)
  point P1 (12.5, -15)
  dimension "d326" = 0.3
  dimension "d327" = 17
  dimension "d328" = 2.5
  dimension "d329" = 2.5
  constraints: 10 end point, 3 centre point, 1 point on line
  measures "d326" distance of L1.start L4.end
  measures "d327" diameter of A0
  measures "d328" diameter of A1
  measures "d329" diameter of A2
extrude "Extrusion48" cut sketch "Sketch50" against normal blind 10 contours A1 | A2
fillet "Fillet1" radius 2 4 edges at (-85, 7.5, -52.6783) (-85, 7.5, -47.6783) (-85, 7.5, 47.6783) (-85, 7.5, 52.6783)
fillet "Fillet2" radius 2 2 edges at (-70, 11.15, 0) (-70, 1.65, 0)
fillet "Fillet3" radius 2 4 edges at (-18.7782, 27.5, -63.6088) (6.2218, 27.5, -63.6088) (6.2218, 27.5, -82.8998) (-18.7782, 27.5, -82.8998)
fillet "Fillet4" radius 2 4 edges at (6.2218, 27.5, 62.8998) (-18.7782, 27.5, 62.8998) (6.2218, 27.5, 82.8998) (-18.7782, 27.5, 82.8998)
fillet "Fillet5" radius 2 4 edges at (82, 27.5, 12.5) (62, 27.5, 12.5) (82, 27.5, -12.5) (62, 27.5, -12.5)
chamfer "Chamfer1" distance 2 angle 45 24 edges at (5.636, 40, 82.314) (-6.2782, 40, 82.8998) (-18.1924, 40, 82.314) (-18.7782, 40, 72.8998) (-18.1924, 40, 63.4856) (-6.2782, 40, 62.8998) (5.636, 40, 63.4856) (6.2218, 40, 72.8998) (82, 40, 0) (81.4142, 40, -11.9142) (72, 40, -12.5) (62.5858, 40, -11.9142) (62, 40, 0) (62.5858, 40, 11.9142) (72, 40, 12.5) (81.4142, 40, 11.9142) (6.2218, 40, -73.2543) (5.636, 40, -82.314) (-6.2782, 40, -82.8998) (-18.1924, 40, -82.314) (-18.7782, 40, -73.2543) (-18.1924, 40, -64.1946) (-6.2782, 40, -63.6088) (5.636, 40, -64.1946)
body "Solid1"
